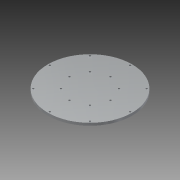
# Autodesk Inventor part: EndCap
Saved by Autodesk Inventor 2015 (Build 190159000, 159)
## iProperties
Created: 2015-09-24
Part Number: EndCap
Material: Generic
Document SubType Name: Modeling
Designer: Stefania
Density: 1 g/cm^3
Appearance: Clear
Author: Stefania
Autodesk Inventor part; units mm, degrees
ref_plane "YZ Plane" through (0, 0, 0) normal (1, 0, 0) x (0, 1, 0)
ref_plane "XZ Plane" through (0, 0, 0) normal (0, 1, 0) x (-1, 0, 0)
ref_plane "XY Plane" through (0, 0, 0) normal (0, 0, 1) x (1, 0, 0)
sketch "Sketch1" plane through (0, 0, 0) normal (0, 0, 1) x (1, 0, 0)
  circle A0 centre (0, 0) radius 83.82
  dimension "d0" = 167.64
  constraints: 1 centre point, 1 coincident
  measures "d0" diameter of A0
extrude "Extrusion1" add sketch "Sketch1" along normal mid plane 5.08
sketch "Sketch2" plane through (0, 0, 2.54) normal (0, 0, 1) x (1, 0, 0)
  circle A0 centre (0, 80.01) radius 1.7526
  circle A1 centre (-56.5756, 56.5756) radius 1.7526
  circle A2 centre (-80.01, 0) radius 1.7526
  circle A3 centre (-56.5756, -56.5756) radius 1.7526
  circle A4 centre (0, -80.01) radius 1.7526
  circle A5 centre (56.5756, -56.5756) radius 1.7526
  circle A6 centre (80.01, 0) radius 1.7526
  circle A7 centre (56.5756, 56.5756) radius 1.7526
  point P0 (0, 0)
  dimension "d3" = 3.5052
  dimension "d6" = 360
  constraints: 8 centre point, 17 other
  measures "d3" diameter of A0
extrude "Extrusion2" cut sketch "Sketch2" against normal through all
sketch "Sketch3" plane through (0, 0, 2.54) normal (0, 0, 1) x (1, 0, 0)
  circle A0 centre (0, 40.9092) radius 1.7526
  circle A1 centre (-28.9272, 28.9272) radius 1.7526
  circle A2 centre (28.9272, 28.9272) radius 1.7526
  circle A3 centre (-40.9092, 0) radius 1.7526
  circle A4 centre (40.9092, 0) radius 1.7526
  circle A5 centre (0, -40.9092) radius 1.7526
  circle A6 centre (-28.9272, -28.9272) radius 1.7526
  circle A7 centre (28.9272, -28.9272) radius 1.7526
  point P0 (0, 0)
  point P1 (0, 0)
  point P2 (-37.0992, 0)
  dimension "d12" = 3.5052
  dimension "d16" = 45
  dimension "d20" = 45
  dimension "d24" = 45
  dimension "d28" = 45
  constraints: 8 centre point, 1 coincident, 1 horizontal alignment, 12 other
  measures "d12" diameter of A0
extrude "Extrusion3" cut sketch "Sketch3" against normal through all
body "Solid1"
